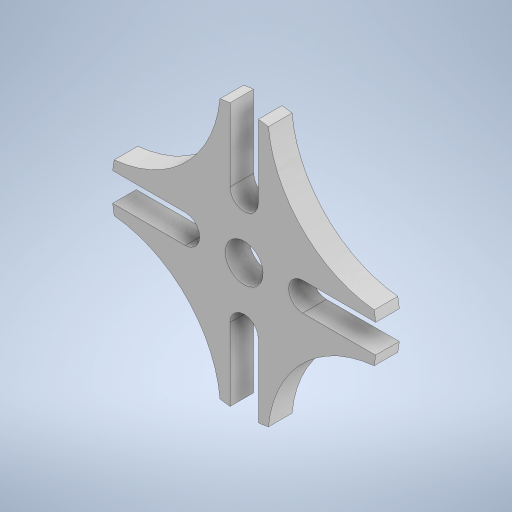
# Autodesk Inventor part: Geneva_driven
Saved by Autodesk Inventor 2024 (Build 280153000, 153)
## iProperties
Created: 2024-01-31
Part Number: Geneva_driven
Material: Generic
Document SubType Name: Modeling
Designer: yogde
Density: 1 g/cm^3
Appearance: Default
Author: yogde
Autodesk Inventor part; units mm, degrees
ref_plane "YZ Plane" through (0, 0, 0) normal (1, 0, 0) x (0, 1, 0)
ref_plane "XZ Plane" through (0, 0, 0) normal (0, 1, 0) x (-1, 0, 0)
ref_plane "XY Plane" through (0, 0, 0) normal (0, 0, 1) x (1, 0, 0)
sketch "Sketch1" plane through (0, 0, 0) normal (0, 0, 1) x (1, 0, 0)
  circle A0 centre (0, 0) radius 28
  dimension "d0" = 56
  constraints: 1 centre point, 1 coincident
  measures "d0" diameter of A0
extrude "Extrusion1" add sketch "Sketch1" along normal blind 5
sketch "Sketch2" plane through (0, 0, 5) normal (0, 0, 1) x (1, 0, 0)
  line L0 (0, 0) -> (30, 0) construction
  line L1 (30, 0) -> (30, 30) construction
  line L2 (30, 30) -> (0, 30) construction
  line L3 (0, 30) -> (0, 0) construction
  circle A0 centre (0, 0) radius 30 construction
  circle A1 centre (30, 30) radius 30 construction
  circle A2 centre (0, 0) radius 12.4264 construction
  circle A3 centre (30, 30) radius 25
  circle A4 centre (0, 0) radius 4
  line L4 (12.4264, 0) -> (30, 0) construction
  line L5 (12.4264, -3) -> (30, -3)
  line L6 (30, 3) -> (12.4264, 3)
  arc A5 (12.4264, 3) -> (12.4264, -3) centre (12.4264, 0) ccw
  arc A6 (30, -3) -> (30, 3) centre (30, 0) ccw
  point P0 (21.2132, 0)
  dimension "d5" = 60
  dimension "d3" = 30
  dimension "d4" = 30
  dimension "d6" = 60
  dimension "d7" = 50
  dimension "d8" = 8
  dimension "d9" = 6
  constraints: 16 end point, 5 centre point, 5 coincident, 4 point on circle, 4 tangent, 3 parallel, 2 horizontal alignment, 2 point on line, 1 horizontal, 1 midpoint, 1 perpendicular, 5 other
  measures "d3" distance of L2.end L1.end
  measures "d4" distance of L1.end L0.end
  measures "d6" diameter of A1
  measures "d7" diameter of A3
  measures "d8" diameter of A4
  measures "d9" diameter of A6
extrude "Extrusion2" cut sketch "Sketch2" against normal blind 5
pattern_circular "Circular Pattern1" count 4 over 360 about axis through (0, 0, 5) along (0, 0, -1) of "Extrusion2"
body "Solid1"
